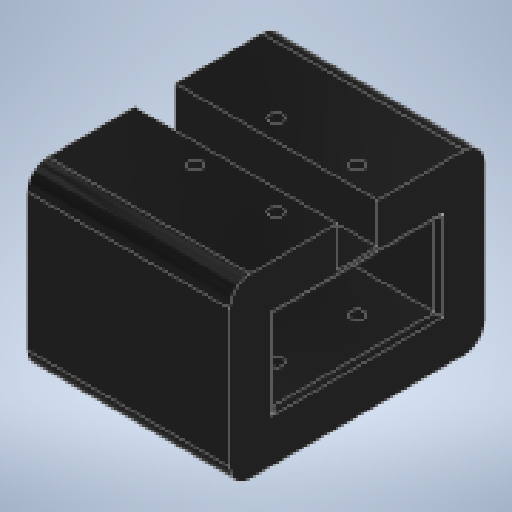
# Autodesk Inventor part: framefixpart1_forearm
Saved by Autodesk Inventor 2024.3 (Build 283343010, 343A)
## iProperties
Created: 2025-05-29
Part Number: framefixpart1_forearm
Material: 一般
Document SubType Name: Modeling
Designer: kshau
Density: 1 g/cm^3
Appearance: 滑らか - 黒
Author: kshau
Autodesk Inventor part; units mm, degrees
ref_plane "YZ Plane" through (0, 0, 0) normal (1, 0, 0) x (0, 1, 0)
ref_plane "XZ Plane" through (0, 0, 0) normal (0, 1, 0) x (-1, 0, 0)
ref_plane "XY Plane" through (0, 0, 0) normal (0, 0, 1) x (1, 0, 0)
sketch "スケッチ1" plane through (0, 0, 0) normal (1, 0, 0) x (0, 1, 0)
  line L0 (0, 0) -> (43.8, 0)
  line L1 (43.8, 0) -> (43.8, -62.8)
  line L2 (43.8, -62.8) -> (0, -62.8)
  line L3 (0, -62.8) -> (0, 0)
  dimension "d0" = 43.8
  dimension "d1" = 62.8
  constraints: 8 end point, 2 parallel, 1 horizontal, 1 perpendicular
  measures "d0" distance of L1.end L2.end
  measures "d1" distance of L0.end L1.end
extrude "押し出し1" add sketch "スケッチ1" along normal blind 50
sketch "スケッチ2" plane through (50, 0, 0) normal (1, 0, 0) x (0, 0, -1)
  line L0 (0, 43.8) -> (0, 0) projected
  line L1 (0, 21.9) -> (62.8, 21.9)
  line L2 (62.8, 0) -> (62.8, 43.8) projected
  line L3 (62.8, 43.8) -> (0, 43.8) projected
  line L4 (31.4, 43.8) -> (31.4, 0)
  line L5 (0, 0) -> (62.8, 0) projected
  line L6 (31.4, 21.9) -> (51.5, 21.9)
  line L7 (51.5, 21.9) -> (51.5, 32)
  line L8 (51.5, 32) -> (31.4, 32)
  line L9 (31.4, 32) -> (31.4, 21.9)
  line L10 (11.3, 21.9) -> (11.3, 32)
  line L11 (11.3, 32) -> (31.4, 32)
  line L12 (51.5, 21.9) -> (51.5, 11.8)
  line L13 (51.5, 11.8) -> (31.4, 11.8)
  line L14 (11.3, 11.8) -> (31.4, 11.8)
  line L15 (11.3, 21.9) -> (11.3, 11.8)
  dimension "d4" = 20.1
  dimension "d5" = 10.1
  constraints: 24 end point, 5 midpoint, 5 symmetric about line, 2 parallel, 1 horizontal, 1 perpendicular
  measures "d4" distance of L7.end L8.end
  measures "d5" distance of L6.end L7.end
extrude "押し出し2" cut sketch "スケッチ2" against normal blind 40 contours L10 L11 L4 L1 | L1 L4 L14 L15 | L8 L7 L1 L4 | L1 L12 L13 L4
sketch "スケッチ3" plane through (0, 43.8, 0) normal (0, 1, 0) x (1, 0, 0)
  line L0 (0, 0) -> (50, 0) projected
  line L1 (10, 0) -> (10, 62.8)
  line L2 (0, 62.8) -> (50, 62.8) projected
  line L3 (0, 62.8) -> (0, 0) projected
  line L4 (0, 31.4) -> (50, 31.4)
  line L5 (50, 0) -> (50, 62.8) projected
  line L6 (10, 41.4) -> (50, 41.4)
  point P0 (20, 41.4)
  point P1 (40, 41.4)
  point P2 (20, 21.4)
  point P3 (40, 21.4)
  dimension "d8" = 10
  dimension "d9" = 10
  dimension "d10" = 10
  dimension "d11" = 20
  constraints: 6 end point, 6 point on line, 2 midpoint, 2 symmetric about line, 1 parallel, 1 vertical
  measures "d8" distance between parallel lines of L3 L1
  measures "d9" distance between parallel lines of L4 L6
  measures "d10" distance from line of L1 point (20, 41.4)
  measures "d11" distance of point (20, 41.4) point (40, 41.4)
hole "穴1" at (20, 43.8, -41.4) at (40, 43.8, -41.4) at (20, 43.8, -21.4) at (40, 43.8, -21.4) direction (0, -1, 0) diameter 3.3 end through all
fillet "フィレット1" radius 5 4 edges at (25, 43.8, 0) (25, 0, 0) (25, 0, -62.8) (25, 43.8, -62.8)
sketch "スケッチ4" plane through (10, 0, 0) normal (1, 0, 0) x (0, 0, -1)
  line L0 (11.3, 11.8) -> (11.3, 32) projected
  line L1 (11.3, 21.9) -> (51.5, 21.9)
  line L2 (51.5, 32) -> (51.5, 11.8) projected
  line L3 (11.3, 32) -> (51.5, 32) projected
  line L4 (31.4, 32) -> (31.4, 11.8)
  line L5 (51.5, 11.8) -> (11.3, 11.8) projected
  point P0 (0, 0)
  point P1 (41.4, 21.9)
  point P2 (21.4, 21.9)
  dimension "d20" = 10
  constraints: 4 end point, 4 midpoint, 1 point on line, 1 symmetric about line
  measures "d20" distance from line of L4 point (41.4, 21.9)
hole "穴2" at (10, 21.9, -41.4) at (10, 21.9, -21.4) direction (-1, 0, 0) diameter 3.3 end through all
fillet "フィレット2" radius 1 4 edges at (50, 21.9, -51.5) (50, 11.8, -31.4) (50, 32, -31.4) (50, 21.9, -11.3)
sketch "スケッチ5" plane through (50, 0, 0) normal (1, 0, 0) x (0, 0, -1)
  line L0 (57.8, 43.8) -> (5, 43.8) projected
  line L1 (31.4, 43.8) -> (31.4, 33)
  line L2 (52.5, 33) -> (10.3, 33) projected
  line L3 (31.4, 43.8) -> (36.4, 43.8)
  line L4 (36.4, 43.8) -> (36.4, 33.8)
  line L5 (36.4, 33.8) -> (31.4, 33.8)
  line L6 (31.4, 33.8) -> (31.4, 43.8)
  line L7 (26.4, 43.8) -> (26.4, 33.8)
  line L8 (26.4, 33.8) -> (31.4, 33.8)
  point P0 (0, 0)
  dimension "d29" = 10
  dimension "d30" = 5
  constraints: 14 end point, 2 midpoint, 2 parallel, 2 symmetric about line, 1 horizontal, 1 perpendicular
  measures "d29" distance of L3.end L4.end
  measures "d30" distance between parallel lines of L1 L4
extrude "押し出し3" cut sketch "スケッチ5" against normal blind 100
